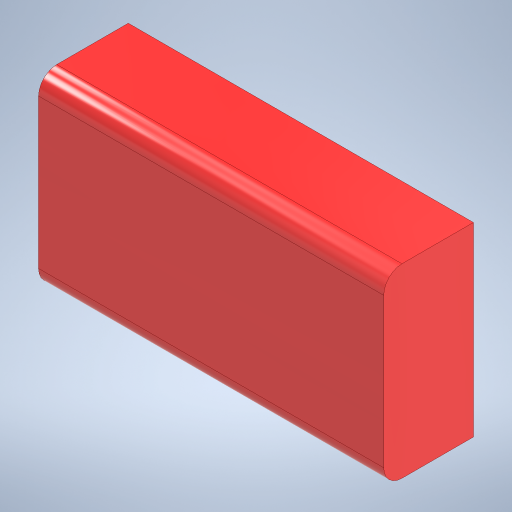
# Autodesk Inventor part: prop_battery
Saved by Autodesk Inventor 2024.2 (Build 282272000, 272)
## iProperties
Created: 2025-03-01
Part Number: prop_battery
Material: Všeobecné
Document SubType Name: Modeling
Designer: hepma_axt67em
Density: 1 g/cm^3
Appearance: Světle červená
Author: hepma_axt67em
Autodesk Inventor part; units mm, degrees
ref_plane "YZ Plane" through (0, 0, 0) normal (1, 0, 0) x (0, 1, 0)
ref_plane "XZ Plane" through (0, 0, 0) normal (0, 1, 0) x (-1, 0, 0)
ref_plane "XY Plane" through (0, 0, 0) normal (0, 0, 1) x (1, 0, 0)
sketch "Náčrt1" plane through (0, 0, 0) normal (0, 0, 1) x (1, 0, 0)
  line L0 (0, 28.56) -> (0, -28.56) projected
  line L1 (-53.06, 0) -> (53.06, 0) projected
  line L2 (-37.9, 20.4) -> (37.9, 20.4)
  line L3 (37.9, 20.4) -> (37.9, -20.4)
  line L4 (37.9, -20.4) -> (-37.9, -20.4)
  line L5 (-37.9, -20.4) -> (-37.9, 20.4)
  point P0 (0, 0)
  dimension "d0" = 75.8
  dimension "d1" = 40.8
  constraints: 8 end point, 2 parallel, 1 horizontal, 1 perpendicular, 2 other
  measures "d0" distance of L3.end L4.end
  measures "d1" distance of L2.end L3.end
extrude "Vysunutí1" add sketch "Náčrt1" along normal blind 19.7
fillet "Zaoblení1" radius 4 2 edges at (0, 20.4, 19.7) (0, -20.4, 19.7)
